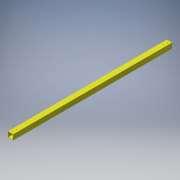
# Autodesk Inventor part: Long Side
Saved by Autodesk Inventor 2017 (Build 210142000, 142)
## iProperties
Created: 2017-01-16
Part Number: Long Side
Material: Aluminum 6061
Document SubType Name: Modeling
Designer: Ben
Density: 2.7 g/cm^3
Appearance: Smooth - Yellow
Mass: 305.739 g
Surface Area: 1430.64 cm^2
Volume: 113.237 cm^3
Author: Ben
Autodesk Inventor part; units mm, degrees
ref_plane "YZ Plane" through (0, 0, 0) normal (1, 0, 0) x (0, 1, 0)
ref_plane "XZ Plane" through (0, 0, 0) normal (0, 1, 0) x (-1, 0, 0)
ref_plane "XY Plane" through (0, 0, 0) normal (0, 0, 1) x (1, 0, 0)
sketch "Sketch1" plane through (0, 0, 0) normal (0, 0, 1) x (1, 0, 0)
  line L0 (0, 0) -> (-11.1125, 0) construction
  line L1 (0, 0) -> (0, 11.1125) construction
  line L2 (-11.1125, 11.1125) -> (11.1125, 11.1125)
  line L3 (11.1125, 11.1125) -> (11.1125, -11.1125)
  line L4 (11.1125, -11.1125) -> (-11.1125, -11.1125)
  line L5 (-11.1125, -11.1125) -> (-11.1125, 11.1125)
  line L6 (-12.7, 12.7) -> (12.7, 12.7)
  line L7 (12.7, 12.7) -> (12.7, -12.7)
  line L8 (12.7, -12.7) -> (-12.7, -12.7)
  line L9 (-12.7, -12.7) -> (-12.7, 12.7)
  line L10 (-11.1125, 0) -> (-12.7, 0) construction
  line L11 (0, 11.1125) -> (0, 12.7) construction
  dimension "d0" = 25.4
  dimension "d1" = 1.5875
  constraints: 24 end point, 4 horizontal, 4 midpoint, 4 parallel, 4 perpendicular, 2 vertical
  measures "d0" distance of L8.end L6.start
  measures "d1" distance of L1.end L11.end
extrude "Extrusion1" add sketch "Sketch1" along normal mid plane 768.35
sketch "Sketch3" plane through (-12.7, -12.7, 384.175) normal (0, -1, 0) x (1, 0, 0)
  line L0 (12.7, -384.175) -> (0, -384.175) construction
  line L1 (0, -768.35) -> (0, 0) construction
  line L2 (12.7, -384.175) -> (12.7, 0) construction
  circle A0 centre (12.7, -9.525) radius 1.5875
  circle A1 centre (12.7, -28.575) radius 1.5875
  line L3 (0, 0) -> (25.4, 0) projected
  circle A2 centre (12.7, -758.825) radius 1.5875
  circle A3 centre (12.7, -739.775) radius 1.5875
  dimension "d9" = 3.175
  dimension "d10" = 9.525
  dimension "d11" = 19.05
  constraints: 4 centre point, 4 end point, 2 point on line, 2 symmetric about line, 1 equal radius, 1 midpoint, 1 parallel, 2 other
  measures "d9" diameter of A0
  measures "d10" distance from line of A0.centre L3
  measures "d11" distance of A1.centre A0.centre
extrude "Extrusion3" cut sketch "Sketch3" against normal through all
body "Solid1"
